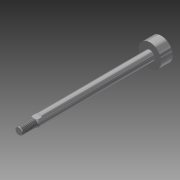
# Autodesk Inventor part: PR_OCG1-3/4x2
Saved by Autodesk Inventor 2016 SP1 (Build 200210100, 210)
## iProperties
Category: PARTsolutions
Company: PHD
Created: 2015-12-03
Part Number: PR_OCG1-3/4x2
Catalog Web Link: www.cadenas.de
Description: OCG1 Piston Rod Assy-OCG1 Cylinder
Vendor: PHD
Document SubType Name: Modeling
Designer: psAdmin
Manufacturer: PHD
Mass: 63.6154 g
Surface Area: 38.0764 cm^2
Volume: 7.95193 cm^3
Density: 8 g/cm^3
Material: Stainless Steel
Appearance: Semi-Polished
PSOL_IDENT_0: {$CADENAS_DATA\23d-libs\phd\cylinders\ocg\parts\ocg_p_r_assy.prj},188 {VTYP=3D},{NB=PR_OCG1-3/4x2},{
PSOL_IDENT_1: LINA=PR_OCG1-3/4x2},{NN=OCG1 Piston Rod Assy},{DATE=20.11.2015 15:31:40},{GEOMDATE=04.02.2015 15:34:
PSOL_IDENT_2: 04},{VERSION=},{LINEID=10},{LINESUBID=-1},{WBVAR=STROKE}  {NB=PR_OCG1-3/4x2},{LINA=PR_OCG1-3/4x2},{K
PSOL_IDENT_3: T=DUMMY},{IDNR=OCG},{DN=1},{SIZE=3/4},{STROKE=2},{A=0.50},{D=0.24},{K=0.157},{KK=1/4-28},{MM=0.315},
PSOL_IDENT_4: {N=0.94},{P=0.47},{R=0.55},{V=0.08},{W=0.50},{KKDIA=0.2500},{STROKE1= '1','2','3','4','5','6','7','8'
PSOL_IDENT_5: },{SIZE1=0.75},{STROKE2=2},{LGTH1=0.709}
NN: OCG1 Piston Rod Assy
NT: OCG1 Cylinder
NB: PR_OCG1-3/4x2
NBSYN: PR_$IDNR.$DN.-$SIZE.x$STROKE.
LINA: PR_OCG1-3/4x2
IDNR: OCG
DN: 1
SIZE: 3/4
STROKE: 2
A: 0.50
D: 0.24
K: 0.157
KK: 1/4-28
MM: 0.315
N: 0.94
P: 0.47
R: 0.55
V: 0.08
W: 0.50
KKDIA: 0.2500
LGTH1: 0.709
SUPPLIER: PHD
ARTICLENO: PR_OCG1-3/4x2
BOMINFO: PR_OCG1-3/4x2
CREATOR: CADENAS GmbH
Title: PR_OCG1-3/4x2
Author: Cadenas PARTsolutions
Comments: OCG1 Cylinder
Autodesk Inventor part; units mm, degrees
sketch "Sketch_1" plane through (0, 0, 0) normal (1, 0, 0) x (0, 1, 0)
  line L0 (0, -106.5721) -> (0, 12.7)
  line L1 (0, 12.7) -> (2.634, 12.7)
  line L2 (2.634, 12.7) -> (3.175, 12.159)
  line L3 (3.175, 12.159) -> (3.175, 0)
  line L4 (3.175, 0) -> (4.0005, -0.8255)
  line L5 (4.0005, -0.8255) -> (4.0005, -97.0471)
  line L6 (4.0005, -97.0471) -> (9.5123, -97.0471)
  line L7 (9.5123, -97.0471) -> (9.5123, -106.5721)
  line L8 (9.5123, -106.5721) -> (0, -106.5721)
  line L9 (0, -106.5721) -> (0, 12.7)
  constraints: 20 end point
revolve "Revolution1" add sketch "Sketch_1" angle 360 about axis through (0, 0, -106.5721) along (0, 0, -1)
thread "Thread1" size "1/4-28 UNF" class "2A" standard "ANSI Unified Screw Threads" full length
sketch "Sketch_2" plane through (0, 0, 0) normal (1, 0, 0) x (0, 1, 0)
  line L0 (6.096, 0) -> (3.048, 0)
  line L1 (3.048, 0) -> (3.048, -3.9878)
  line L2 (3.048, -3.9878) -> (6.096, -7.0358)
  line L3 (6.096, -7.0358) -> (6.096, 0)
  constraints: 8 end point
extrude "Extrusion1" cut sketch "Sketch_2" along normal mid plane 16.002
sketch "Sketch_3" plane through (0, 0, 0) normal (1, 0, 0) x (0, 1, 0)
  line L0 (-6.096, 0) -> (-6.096, -7.0358)
  line L1 (-6.096, -7.0358) -> (-3.048, -3.9878)
  line L2 (-3.048, -3.9878) -> (-3.048, 0)
  line L3 (-3.048, 0) -> (-6.096, 0)
  constraints: 8 end point
extrude "Extrusion2" cut sketch "Sketch_3" along normal mid plane 16.002
ref_plane "conn_XY" through (0, 0, 0) normal (0, 0, -1) x (1, 0, 0)
ref_plane "conn_YZ" through (0, 0, 0) normal (1, 0, 0) x (0, -1, 0)
ref_plane "conn_ZX" through (0, 0, 0) normal (0, -1, 0) x (0, 0, -1)
body "Solid1"
